Autodesk Fusion 360 part; units mm, degrees
(part 7 of 7)
  spline S39 degree 5 poles (-10.5599, 3.0803) (-10.5564, 3.0764) (-10.5492, 3.0687) (-10.5385, 3.057) (-10.5242, 3.0416) (-10.5063, 3.0224) (-10.4883, 3.0034) (-10.4703, 2.9844) (-10.4522, 2.9656) (-10.434, 2.9469) (-10.4158, 2.9283) (-10.3975, 2.9098) (-10.3791, 2.8915) (-10.3607, 2.8732) (-10.3422, 2.8551) (-10.3237, 2.8371) (-10.3051, 2.8193) (-10.2864, 2.8015) (-10.2677, 2.7839) (-10.249, 2.7664) (-10.2301, 2.7491) (-10.2112, 2.7318) (-10.1923, 2.7147) (-10.1733, 2.6977) (-10.1542, 2.6809) (-10.1351, 2.6642) (-10.1159, 2.6476) (-10.0966, 2.6311) (-10.0773, 2.6148) (-10.058, 2.5986) (-10.0386, 2.5826) (-10.0191, 2.5667) (-9.9995, 2.5509) (-9.9799, 2.5353) (-9.9603, 2.5198) (-9.9406, 2.5045) (-9.9208, 2.4893) (-9.901, 2.4743) (-9.8811, 2.4594) (-9.8611, 2.4446) (-9.8411, 2.43) (-9.821, 2.4156) (-9.8009, 2.4014) (-9.7807, 2.3873) (-9.7605, 2.3733) (-9.7402, 2.3595) (-9.7198, 2.3459) (-9.6994, 2.3325) (-9.6789, 2.3192) (-9.6584, 2.3061) (-9.6378, 2.2932) (-9.6171, 2.2805) (-9.5964, 2.2679) (-9.5755, 2.2556) (-9.5547, 2.2435) (-9.5338, 2.2315) (-9.5128, 2.2198) (-9.4917, 2.2082) (-9.4706, 2.1968) (-9.4495, 2.1856) (-9.4282, 2.1747) (-9.4069, 2.1641) (-9.3855, 2.1539) (-9.3639, 2.1439) (-9.3423, 2.1342) (-9.3207, 2.1248) (-9.299, 2.1154) (-9.2772, 2.1063) (-9.2554, 2.0974) (-9.2335, 2.0889) (-9.2115, 2.0811) (-9.1936, 2.0755) (-9.1801, 2.0719) (-9.171, 2.0697) (-9.1664, 2.0687) knots -1 -1 -1 -1 -1 -1 -0.98571429 -0.97142857 -0.95714286 -0.94285714 -0.92857143 -0.91428571 -0.9 -0.88571429 -0.87142857 -0.85714286 -0.84285714 -0.82857143 -0.81428571 -0.8 -0.78571429 -0.77142857 -0.75714286 -0.74285714 -0.72857143 -0.71428571 -0.7 -0.68571429 -0.67142857 -0.65714286 -0.64285714 -0.62857143 -0.61428571 -0.6 -0.58571429 -0.57142857 -0.55714286 -0.54285714 -0.52857143 -0.51428571 -0.5 -0.48571429 -0.47142857 -0.45714286 -0.44285714 -0.42857143 -0.41428571 -0.4 -0.38571429 -0.37142857 -0.35714286 -0.34285714 -0.32857143 -0.31428571 -0.3 -0.28571429 -0.27142857 -0.25714286 -0.24285714 -0.22857143 -0.21428571 -0.2 -0.18571429 -0.17142857 -0.15714286 -0.14285714 -0.12857143 -0.11428571 -0.1 -0.08571429 -0.07142857 -0.05714286 -0.04285714 -0.02857143 -0.01428571 0 0 0 0 0 0
  line L39 (-9.1664, 2.0687) -> (-8.9139, 2.0117)
  arc A79 (-8.6853, 1.6627) -> (-8.9139, 2.0117) centre (-8.9799, 1.7191) ccw
  circle A80 centre (0, 0) radius 2.6
sketch "Base Circle (3)" plane through (0, 0, 0) normal (0, 0, 1) x (1, 0, 0)
  circle A0 centre (0, 0) radius 13.2645
  circle A1 centre (0, 0) radius 3.5
  circle A2 centre (0, 10.2645) radius 2
  line L0 (0, 13.2645) -> (0, -13.2645) construction
  circle A3 centre (-6.0333, 8.3042) radius 2
  circle A4 centre (-9.7621, 3.1719) radius 2
  circle A5 centre (-9.7621, -3.1719) radius 2
  circle A6 centre (-6.0333, -8.3042) radius 2
  circle A7 centre (0, -10.2645) radius 2
  circle A8 centre (6.0333, -8.3042) radius 2
  circle A9 centre (9.7621, -3.1719) radius 2
  circle A10 centre (9.7621, 3.1719) radius 2
  circle A11 centre (6.0333, 8.3042) radius 2
  dimension "d9" = 4
  dimension "d10" = 3
  dimension "d12" = 360
  constraint coincident A0 L0.start
  constraint coincident A0 L0.end
  constraint vertical L0
  constraint coincident A0.centre L0
  constraint coincident A2.centre L0
  measures "d9" diameter of A2
  measures "d10" distance of A2.centre L0.start
extrude "Extrude1" [suppressed]
sketch "Gear Tooth (3)" plane through (0, 0, 0) normal (0, 0, 1) x (1, 0, 0)
  spline S0 degree 5 poles (14.0339, -1.3152) (14.0409, -1.3159) (14.055, -1.317) (14.076, -1.3181) (14.1042, -1.3186) (14.1395, -1.3177) (14.1748, -1.3157) (14.2101, -1.3131) (14.2455, -1.3102) (14.2809, -1.307) (14.3163, -1.3035) (14.3517, -1.2998) (14.3871, -1.2956) (14.4226, -1.2909) (14.458, -1.2856) (14.4935, -1.2799) (14.529, -1.2738) (14.5644, -1.2674) (14.5999, -1.2606) (14.6354, -1.2536) (14.6708, -1.2463) (14.7063, -1.2386) (14.7418, -1.2307) (14.7772, -1.2225) (14.8127, -1.2139) (14.8481, -1.2051) (14.8836, -1.1959) (14.919, -1.1865) (14.9544, -1.1768) (14.9898, -1.1668) (15.0252, -1.1566) (15.0606, -1.1461) (15.0959, -1.1354) (15.1313, -1.1244) (15.1666, -1.1131) (15.202, -1.1016) (15.2373, -1.0899) (15.2726, -1.0779) (15.3078, -1.0656) (15.3431, -1.0532) (15.3783, -1.0405) (15.4135, -1.0275) (15.4487, -1.0144) (15.4839, -1.001) (15.519, -0.9874) (15.5542, -0.9735) (15.5893, -0.9594) (15.6244, -0.9452) (15.6594, -0.9307) (15.6944, -0.9159) (15.7294, -0.901) (15.7644, -0.8859) (15.7994, -0.8705) (15.8343, -0.8549) (15.8692, -0.8392) (15.904, -0.8232) (15.9389, -0.807) (15.9737, -0.7906) (16.0085, -0.774) (16.0432, -0.7572) (16.0779, -0.7402) (16.1126, -0.723) (16.1472, -0.7056) (16.1819, -0.6881) (16.2164, -0.6703) (16.251, -0.6523) (16.2855, -0.6341) (16.32, -0.6158) (16.3544, -0.5972) (16.3888, -0.5785) (16.4232, -0.5595) (16.4506, -0.5442) (16.4712, -0.5327) (16.4849, -0.525) (16.4918, -0.5211) knots 0 0 0 0 0 0 0.01428571 0.02857143 0.04285714 0.05714286 0.07142857 0.08571429 0.1 0.11428571 0.12857143 0.14285714 0.15714286 0.17142857 0.18571429 0.2 0.21428571 0.22857143 0.24285714 0.25714286 0.27142857 0.28571429 0.3 0.31428571 0.32857143 0.34285714 0.35714286 0.37142857 0.38571429 0.4 0.41428571 0.42857143 0.44285714 0.45714286 0.47142857 0.48571429 0.5 0.51428571 0.52857143 0.54285714 0.55714286 0.57142857 0.58571429 0.6 0.61428571 0.62857143 0.64285714 0.65714286 0.67142857 0.68571429 0.7 0.71428571 0.72857143 0.74285714 0.75714286 0.77142857 0.78571429 0.8 0.81428571 0.82857143 0.84285714 0.85714286 0.87142857 0.88571429 0.9 0.91428571 0.92857143 0.94285714 0.95714286 0.97142857 0.98571429 1 1 1 1 1 1
  spline S1 degree 5 poles (14.0339, 1.3152) (14.0409, 1.3159) (14.055, 1.317) (14.076, 1.3181) (14.1042, 1.3186) (14.1395, 1.3177) (14.1748, 1.3157) (14.2101, 1.3131) (14.2455, 1.3102) (14.2809, 1.307) (14.3163, 1.3035) (14.3517, 1.2998) (14.3871, 1.2956) (14.4226, 1.2909) (14.458, 1.2856) (14.4935, 1.2799) (14.529, 1.2738) (14.5644, 1.2674) (14.5999, 1.2606) (14.6354, 1.2536) (14.6708, 1.2463) (14.7063, 1.2386) (14.7418, 1.2307) (14.7772, 1.2225) (14.8127, 1.2139) (14.8481, 1.2051) (14.8836, 1.1959) (14.919, 1.1865) (14.9544, 1.1768) (14.9898, 1.1668) (15.0252, 1.1566) (15.0606, 1.1461) (15.0959, 1.1354) (15.1313, 1.1244) (15.1666, 1.1131) (15.202, 1.1016) (15.2373, 1.0899) (15.2726, 1.0779) (15.3078, 1.0656) (15.3431, 1.0532) (15.3783, 1.0405) (15.4135, 1.0275) (15.4487, 1.0144) (15.4839, 1.001) (15.519, 0.9874) (15.5542, 0.9735) (15.5893, 0.9594) (15.6244, 0.9452) (15.6594, 0.9307) (15.6944, 0.9159) (15.7294, 0.901) (15.7644, 0.8859) (15.7994, 0.8705) (15.8343, 0.8549) (15.8692, 0.8392) (15.904, 0.8232) (15.9389, 0.807) (15.9737, 0.7906) (16.0085, 0.774) (16.0432, 0.7572) (16.0779, 0.7402) (16.1126, 0.723) (16.1472, 0.7056) (16.1819, 0.6881) (16.2164, 0.6703) (16.251, 0.6523) (16.2855, 0.6341) (16.32, 0.6158) (16.3544, 0.5972) (16.3888, 0.5785) (16.4232, 0.5595) (16.4506, 0.5442) (16.4712, 0.5327) (16.4849, 0.525) (16.4918, 0.5211) knots 0 0 0 0 0 0 0.01428571 0.02857143 0.04285714 0.05714286 0.07142857 0.08571429 0.1 0.11428571 0.12857143 0.14285714 0.15714286 0.17142857 0.18571429 0.2 0.21428571 0.22857143 0.24285714 0.25714286 0.27142857 0.28571429 0.3 0.31428571 0.32857143 0.34285714 0.35714286 0.37142857 0.38571429 0.4 0.41428571 0.42857143 0.44285714 0.45714286 0.47142857 0.48571429 0.5 0.51428571 0.52857143 0.54285714 0.55714286 0.57142857 0.58571429 0.6 0.61428571 0.62857143 0.64285714 0.65714286 0.67142857 0.68571429 0.7 0.71428571 0.72857143 0.74285714 0.75714286 0.77142857 0.78571429 0.8 0.81428571 0.82857143 0.84285714 0.85714286 0.87142857 0.88571429 0.9 0.91428571 0.92857143 0.94285714 0.95714286 0.97142857 0.98571429 1 1 1 1 1 1
  arc A0 (16.4918, -0.5211) -> (16.4918, 0.5211) centre (0, 0) ccw
  line L0 (13.1967, -1.2368) -> (14.0339, -1.3152)
  line L1 (13.1967, 1.2368) -> (14.0339, 1.3152)
  line L2 (13.1967, -1.2368) -> (13.1967, 1.2368)
  point P0 (14.2066, -1.3133)
  point P1 (14.3806, -1.2963)
  point P2 (14.5555, -1.2689)
  point P3 (14.7309, -1.2331)
  point P4 (14.9068, -1.1897)
  point P5 (15.083, -1.1393)
  point P6 (15.2594, -1.0823)
  point P7 (15.4358, -1.0191)
  point P8 (15.6123, -0.95)
  point P9 (15.7887, -0.8751)
  point P10 (15.965, -0.7947)
  point P11 (16.1409, -0.7088)
  point P12 (16.3166, -0.6175)
  point P13 (14.2066, 1.3133)
  point P14 (14.3806, 1.2963)
  point P15 (14.5555, 1.2689)
  point P16 (14.7309, 1.2331)
  point P17 (14.9068, 1.1897)
  point P18 (15.083, 1.1393)
  point P19 (15.2594, 1.0823)
  point P20 (15.4358, 1.0191)
  point P21 (15.6123, 0.95)
  point P22 (15.7887, 0.8751)
  point P23 (15.965, 0.7947)
  point P24 (16.1409, 0.7088)
  point P25 (16.3166, 0.6175)
extrude "Extrude2" [suppressed]
fillet "Fillet1" [suppressed]
pattern_circular "C-Pattern1" [suppressed]
sketch "Diametrial Pitch Circle (3)" plane through (0, 0, 0) normal (0, 0, 1) x (1, 0, 0)
  circle A0 centre (0, 0) radius 15 construction
extrude "Extrude3" [suppressed]
named bodies: "Spur Gear (20 teeth)", "Spur Gear (25 teeth)"
